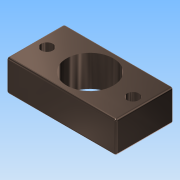
# Autodesk Inventor part: держатель валов
Saved by Autodesk Inventor 2017 (Build 210142000, 142)
## iProperties
Part Number: держатель валов
Material: Типовые
Document SubType Name: Modeling
Designer: Max
Mass: 2.28659 g
Surface Area: 16.6763 cm^2
Volume: 2.28659 cm^3
Density: 1 g/cm^3
Appearance: Оружейный металл — антик — полированный
Author: Max
Autodesk Inventor part; units mm, degrees
ref_plane "YZ Plane" through (0, 0, 0) normal (1, 0, 0) x (0, 1, 0)
ref_plane "XZ Plane" through (0, 0, 0) normal (0, 1, 0) x (-1, 0, 0)
ref_plane "XY Plane" through (0, 0, 0) normal (0, 0, 1) x (1, 0, 0)
sketch "Эскиз1" plane through (0, 0, 0) normal (0, 0, 1) x (1, 0, 0)
  circle A0 centre (0, 0) radius 6
  circle A1 centre (-11, 0) radius 1.5
  circle A2 centre (11, 0) radius 1.5
  line L0 (14, 7.4) -> (-14, 7.4)
  line L1 (-14, 7.4) -> (-14, -7.4)
  line L2 (-14, -7.4) -> (14, -7.4)
  line L3 (14, -7.4) -> (14, 7.4)
  line L4 (14, 7.4) -> (-14, -7.4) construction
  line L5 (-14, 7.4) -> (14, -7.4) construction
  dimension "d0" = 12
  dimension "d1" = 3
  dimension "d2" = 3
  dimension "d3" = 11
  dimension "d4" = 11
  dimension "d5" = 28
  dimension "d6" = 14.8
  constraints: 12 end point, 3 centre point, 2 midpoint, 2 parallel, 1 coincident, 1 horizontal, 1 perpendicular
  measures "d0" diameter of A0
  measures "d1" diameter of A1
  measures "d2" diameter of A2
  measures "d3" distance of point (0, 0) A1.centre
  measures "d4" distance of point (0, 0) A2.centre
  measures "d5" distance between parallel lines of L3 L1
  measures "d6" distance between parallel lines of L0 L2
extrude "Выдавливание1" add sketch "Эскиз1" along normal blind 8
fillet "Сопряжение1" radius 0.5 12 edges at (-14, 7.4, 4) (14, -7.4, 4) (-14, -7.4, 4) (14, 7.4, 4) (0, 7.4, 0) (-14, 0, 0) (0, -7.4, 0) (14, 0, 0) (14, 0, 8) (0, 7.4, 8) (0, -7.4, 8) (-14, 0, 8)
